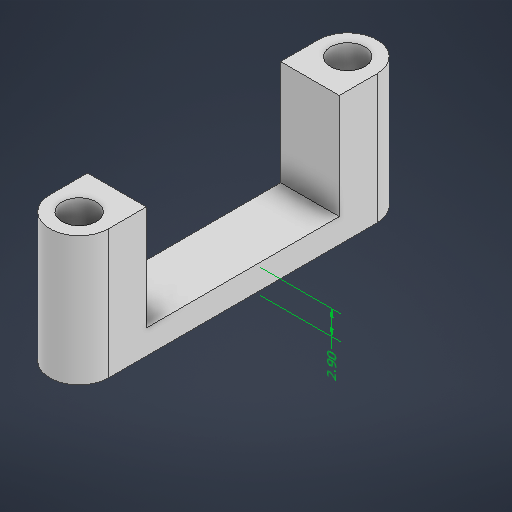
# Autodesk Inventor part: Micro_servo_frame_2
Saved by Autodesk Inventor 2026.1 (Build 301233020, 233B)
## iProperties
Created: 2025-10-15
Part Number: Micro_servo_frame_2
Material: Generic
Document SubType Name: Modeling
Designer: Asus
Density: 1 g/cm^3
Appearance: Default
Author: Asus
Autodesk Inventor part; units mm, degrees
ref_plane "YZ Plane" through (0, 0, 0) normal (1, 0, 0) x (0, 1, 0)
ref_plane "XZ Plane" through (0, 0, 0) normal (0, 1, 0) x (-1, 0, 0)
ref_plane "XY Plane" through (0, 0, 0) normal (0, 0, 1) x (1, 0, 0)
sketch "Sketch1" plane through (0, 0, 0) normal (0, 1, 0) x (-1, 0, 0)
  line L0 (0, 0) -> (0, -32) construction
  line L1 (-3.5, 0) -> (-3.5, -32)
  line L2 (3.5, -32) -> (3.5, 0)
  arc A0 (3.5, 0) -> (-3.5, 0) centre (0, 0) ccw
  arc A1 (-3.5, -32) -> (3.5, -32) centre (0, -32) ccw
  circle A2 centre (0, 0) radius 2.05
  circle A3 centre (0, -32) radius 2.05
  circle A4 centre (0, 0) radius 3.5 construction
  line L3 (-3.5, -4.5) -> (3.5, -4.5)
  line L4 (3.5, -4.5) -> (3.5, -27.5)
  line L5 (3.5, -27.5) -> (-3.5, -27.5)
  line L6 (-3.5, -27.5) -> (-3.5, -4.5)
  line L7 (3.5, -3) -> (-3.5, -3)
  line L8 (3.5, -29) -> (-3.5, -29)
  point P0 (0, -16)
  point P1 (3.5, -16)
  dimension "d0" = 32
  dimension "d1" = 7
  dimension "d2" = 4.1
  dimension "d3" = 4.1
  dimension "d4" = 7
  dimension "d5" = 7
  dimension "d6" = 23
  dimension "d7" = 1.5
  dimension "d8" = 1.5
  constraints: 20 end point, 5 centre point, 4 point on circle, 4 point on line, 4 tangent, 3 coincident, 3 midpoint, 3 parallel, 3 perpendicular, 1 horizontal, 1 vertical
  measures "d0" distance of L0.start L0.end
  measures "d1" diameter of A1
  measures "d2" diameter of A2
  measures "d3" diameter of A3
  measures "d4" diameter of A4
  measures "d5" distance of L4.end L5.end
  measures "d6" distance of L3.end L4.end
  measures "d7" distance between parallel lines of L3 L7
  measures "d8" distance between parallel lines of L8 L5
extrude "Extrusion1" add sketch "Sketch1" along normal blind 14.5
sketch "Sketch3" plane through (0, 14.5, 0) normal (0, 1, 0) x (1, 0, 0)
  line L0 (-3.5, 32) -> (-3.5, 0) projected
  line L1 (-3.5, 4.5) -> (3.5, 4.5)
  line L2 (3.5, 4.5) -> (3.5, 27.5)
  line L3 (3.5, 27.5) -> (-3.5, 27.5)
  line L4 (-3.5, 27.5) -> (-3.5, 4.5)
  point P0 (0, 0)
  point P1 (-3.5, 16)
  dimension "d15" = 7
  dimension "d16" = 23
  constraints: 8 end point, 2 midpoint, 2 parallel, 1 horizontal, 1 perpendicular, 1 point on line
  measures "d15" distance of L3.end L2.end
  measures "d16" distance of L2.end L1.end
extrude "Extrusion2" cut sketch "Sketch3" against normal blind 12.5
sketch "Sketch5" plane through (0, 0, 0) normal (0, -1, 0) x (1, 0, 0)
  line L0 (0, 0) -> (0, -32) construction
  line L1 (-3.5, 0) -> (-3.5, -32)
  line L2 (3.5, -32) -> (3.5, 0)
  arc A0 (3.5, 0) -> (-3.5, 0) centre (0, 0) ccw
  arc A1 (-3.5, -32) -> (3.5, -32) centre (0, -32) ccw
  circle A2 centre (0, 0) radius 2.05
  circle A3 centre (0, -32) radius 2.05
  circle A4 centre (0, 0) radius 3.5 construction
  line L3 (-3.5, -4.5) -> (3.5, -4.5)
  line L4 (3.5, -4.5) -> (3.5, -27.5)
  line L5 (3.5, -27.5) -> (-3.5, -27.5)
  line L6 (-3.5, -27.5) -> (-3.5, -4.5)
  line L7 (3.5, -3) -> (-3.5, -3)
  line L8 (3.5, -29) -> (-3.5, -29)
  point P0 (0, -16)
  point P1 (3.5, -16)
  dimension "d22" = 32
  dimension "d23" = 7
  dimension "d24" = 4.1
  dimension "d25" = 4.1
  dimension "d26" = 7
  dimension "d27" = 7
  dimension "d28" = 23
  dimension "d29" = 1.5
  dimension "d30" = 1.5
  constraints: 20 end point, 5 centre point, 4 coincident, 4 point on circle, 4 point on line, 4 tangent, 3 midpoint, 3 parallel, 3 perpendicular, 1 horizontal, 1 vertical
  measures "d22" distance of L0.start L0.end
  measures "d23" diameter of A1
  measures "d24" diameter of A2
  measures "d25" diameter of A3
  measures "d26" diameter of A4
  measures "d27" distance of L4.end L5.end
  measures "d28" distance of L3.end L4.end
  measures "d29" distance between parallel lines of L3 L7
  measures "d30" distance between parallel lines of L8 L5
extrude "Extrusion3" add sketch "Sketch5" along normal blind 0.9
body "Solid1"
